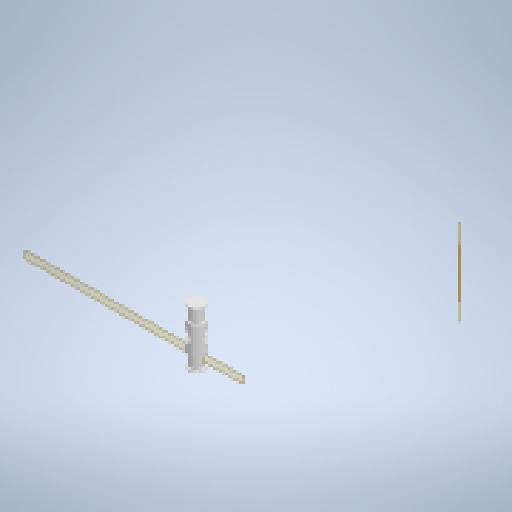
# Autodesk Inventor part: nitR2
Saved by Autodesk Inventor 2025 (Build 290162000, 162)
## iProperties
Created: 2025-02-05
Part Number: nitR2
Material: Generic
Document SubType Name: Modeling
Designer: piotr
Density: 1 g/cm^3
Appearance: Default
Author: piotr
Autodesk Inventor part; units mm, degrees
ref_plane "YZ Plane" through (0, 0, 0) normal (1, 0, 0) x (0, 1, 0)
ref_plane "XZ Plane" through (0, 0, 0) normal (0, 1, 0) x (-1, 0, 0)
ref_plane "XY Plane" through (0, 0, 0) normal (0, 0, 1) x (1, 0, 0)
ref_plane "Work Plane1" through (0, 0, 0) normal (0, 0, 1) x (1, 0, 0)
sketch "Sketch1" plane through (0, 0, 0) normal (0, 0, 1) x (1, 0, 0)
  line L0 (-25.8244, 0) -> (-44.3244, 0) projected
  line L1 (-25.8244, 0) -> (-44.3244, 0) projected
  line L2 (-25.8244, 0) -> (-25.8244, -10)
  line L3 (-25.8244, -10) -> (-22.8244, -10)
  line L4 (-22.8244, -10) -> (-22.8244, -12)
  line L5 (-22.8244, -12) -> (-47.3244, -12)
  line L6 (-47.3244, -12) -> (-47.3244, -10)
  line L7 (-47.3244, -10) -> (-44.3244, -10)
  line L8 (-44.3244, -10) -> (-44.3244, 10)
  line L9 (-44.3244, 10) -> (-47.3244, 10)
  line L10 (-47.3244, 10) -> (-47.3244, 50)
  line L11 (-22.8244, 50) -> (-22.8244, 10)
  line L12 (-22.8244, 10) -> (-25.8244, 10)
  line L13 (-25.8244, 10) -> (-25.8244, 0)
  line L14 (-35.0744, 74.414) -> (-35.0744, -25.586)
  line L15 (-22.8244, 50) -> (-25.8244, 50)
  line L16 (-25.8244, 50) -> (-25.8244, 70)
  line L17 (-25.8244, 70) -> (-22.8244, 70)
  line L18 (-22.8244, 70) -> (-22.8244, 72)
  line L19 (-22.8244, 72) -> (-47.3244, 72)
  line L20 (-47.3244, 72) -> (-47.3244, 70)
  line L21 (-47.3244, 70) -> (-44.3244, 70)
  line L22 (-44.3244, 70) -> (-44.3244, 50)
  line L23 (-44.3244, 50) -> (-47.3244, 50)
  point P0 (0, 0)
  point P1 (-35.0744, 0)
  point P2 (-35.0744, -12)
  point P3 (-44.3244, 0)
  point P4 (-35.0744, 72)
  dimension "d0" = 3
  dimension "d1" = 10
  dimension "d2" = 2
  dimension "d3" = 24.5
  dimension "d4" = 2
  dimension "d5" = 3
  dimension "d6" = 20
  dimension "d8" = 40
  dimension "d18" = 24.5
  dimension "d22" = 100
  constraints: 44 end point, 12 equal length, 11 perpendicular, 7 vertical, 2 horizontal, 1 midpoint, 1 point on line
  measures "d0" distance of L2.end L3.end
  measures "d1" distance of L0.start L2.end
  measures "d2" distance of L3.end L4.end
  measures "d3" distance of L4.end L5.end
  measures "d4" distance of L5.end L6.end
  measures "d5" distance of L6.end L7.end
  measures "d6" distance of L7.end L8.end
  measures "d8" distance of L9.end L10.end
  measures "d18" distance between parallel lines of L10 L11
  measures "d22" distance of L14.start L14.end
revolve "Revolution1" add sketch "Sketch1" angle 360 about axis through (-35.0744, 74.414, 0) along (0, -1, 0) contours L2 L3 L4 L5 L14 L0 | L0 L14 L19 L18 L17 L16 L15 L11 L12 L13
ref_plane "Work Plane2" through (81.744, 30, -281.1346) normal (-0.7042, 0, 0.71) x (0.71, 0, 0.7042)
sketch "Sketch3" plane through (81.744, 30, -281.1346) normal (-0.7042, 0, 0.71) x (0.71, 0, 0.7042)
  line L0 (102.7895, 20) -> (127.2895, 20) projected
  line L1 (102.7895, -20) -> (127.2895, -20) projected
  line L2 (127.2895, 20) -> (102.7895, -20)
  circle A0 centre (115.0395, 0) radius 10
  point P0 (139.9419, -30)
  dimension "d26" = 20
  constraints: 2 end point, 1 centre point, 1 midpoint
  measures "d26" diameter of A0
extrude "Extrusion2" cut sketch "Sketch3" along normal blind 500
body "Solid1"
